Autodesk Fusion 360 part; units mm, degrees
(part 8 of 9)
  spline S368 degree 3 poles (50.2293, -43.6015) (51.1181, -43.6015) (51.7507, -43.8671) (52.1258, -44.3973) knots 0 0 0 0 1 1 1 1
  spline S369 degree 3 poles (52.1258, -44.3973) (52.346, -44.7105) (52.4566, -45.0722) (52.4566, -45.4825) knots 0 0 0 0 1 1 1 1
  spline S370 degree 3 poles (52.4566, -45.4825) (52.4566, -45.961) (52.3201, -46.3538) (52.0483, -46.6607) knots 0 0 0 0 1 1 1 1
  spline S371 degree 3 poles (52.0483, -46.6607) (51.9067, -46.823) (51.7042, -46.9708) (51.4385, -47.1052) knots 0 0 0 0 1 1 1 1
  spline S372 degree 3 poles (51.4385, -47.1052) (51.8282, -47.253) (52.1186, -47.4204) (52.3119, -47.6064) knots 0 0 0 0 1 1 1 1
  spline S373 degree 3 poles (52.3119, -47.6064) (52.6529, -47.9372) (52.8235, -48.394) (52.8235, -48.9758) knots 0 0 0 0 1 1 1 1
  spline S374 degree 3 poles (52.8235, -48.9758) (52.8235, -49.4647) (52.6705, -49.9081) (52.3635, -50.3039) knots 0 0 0 0 1 1 1 1
  spline S375 degree 3 poles (52.3635, -50.3039) (51.9057, -50.8961) (51.1771, -51.1928) (50.1776, -51.1928) knots 0 0 0 0 1 1 1 1
  line L781 (50.1776, -51.1928) -> (46.9685, -51.1928)
  line L782 (46.9685, -51.1928) -> (46.9685, -43.6015)
  line L783 (63.7613, -43.6015) -> (69.2958, -43.6015)
  line L784 (69.2958, -43.6015) -> (69.2958, -44.5317)
  line L785 (69.2958, -44.5317) -> (64.7638, -44.5317)
  line L786 (64.7638, -44.5317) -> (64.7638, -46.8364)
  line L787 (64.7638, -46.8364) -> (68.9548, -46.8364)
  line L788 (68.9548, -46.8364) -> (68.9548, -47.7149)
  line L789 (68.9548, -47.7149) -> (64.7638, -47.7149)
  line L790 (64.7638, -47.7149) -> (64.7638, -50.2884)
  line L791 (64.7638, -50.2884) -> (69.3734, -50.2884)
  line L792 (69.3734, -50.2884) -> (69.3734, -51.1928)
  line L793 (69.3734, -51.1928) -> (63.7613, -51.1928)
  line L794 (63.7613, -51.1928) -> (63.7613, -43.6015)
  line L795 (80.0394, -43.6015) -> (81.2538, -43.6015)
  line L796 (81.2538, -43.6015) -> (85.0882, -49.751)
  line L797 (85.0882, -49.751) -> (85.0882, -43.6015)
  line L798 (85.0882, -43.6015) -> (86.0648, -43.6015)
  line L799 (86.0648, -43.6015) -> (86.0648, -51.1928)
  line L800 (86.0648, -51.1928) -> (84.9125, -51.1928)
  line L801 (84.9125, -51.1928) -> (81.0212, -45.0484)
  line L802 (81.0212, -45.0484) -> (81.0212, -51.1928)
  line L803 (81.0212, -51.1928) -> (80.0394, -51.1928)
  line L804 (80.0394, -51.1928) -> (80.0394, -43.6015)
  line L805 (-86.2575, -62.1017) -> (-80.7229, -62.1017)
  line L806 (-80.7229, -62.1017) -> (-80.7229, -63.0318)
  line L807 (-80.7229, -63.0318) -> (-85.2549, -63.0318)
  line L808 (-85.2549, -63.0318) -> (-85.2549, -65.3366)
  line L809 (-85.2549, -65.3366) -> (-81.064, -65.3366)
  line L810 (-81.064, -65.3366) -> (-81.064, -66.2151)
  line L811 (-81.064, -66.2151) -> (-85.2549, -66.2151)
  line L812 (-85.2549, -66.2151) -> (-85.2549, -68.7886)
  line L813 (-85.2549, -68.7886) -> (-80.6454, -68.7886)
  line L814 (-80.6454, -68.7886) -> (-80.6454, -69.6929)
  line L815 (-80.6454, -69.6929) -> (-86.2575, -69.6929)
  line L816 (-86.2575, -69.6929) -> (-86.2575, -62.1017)
  line L817 (-69.1009, -62.1017) -> (-68.0725, -62.1017)
  line L818 (-68.0725, -62.1017) -> (-68.0725, -68.7886)
  line L819 (-68.0725, -68.7886) -> (-64.2278, -68.7886)
  line L820 (-64.2278, -68.7886) -> (-64.2278, -69.6929)
  line L821 (-64.2278, -69.6929) -> (-69.1009, -69.6929)
  line L822 (-69.1009, -69.6929) -> (-69.1009, -62.1017)
  line L823 (-52.6233, -62.1017) -> (-47.3575, -62.1017)
  line L824 (-47.3575, -62.1017) -> (-47.3575, -63.0318)
  line L825 (-47.3575, -63.0318) -> (-51.595, -63.0318)
  line L826 (-51.595, -63.0318) -> (-51.595, -65.3366)
  line L827 (-51.595, -65.3366) -> (-47.8691, -65.3366)
  line L828 (-47.8691, -65.3366) -> (-47.8691, -66.2409)
  line L829 (-47.8691, -66.2409) -> (-51.595, -66.2409)
  line L830 (-51.595, -66.2409) -> (-51.595, -69.6929)
  line L831 (-51.595, -69.6929) -> (-52.6233, -69.6929)
  line L832 (-52.6233, -69.6929) -> (-52.6233, -62.1017)
  line L833 (-35.7499, -62.1017) -> (-33.5692, -68.5664)
  line L834 (-33.5692, -68.5664) -> (-31.4143, -62.1017)
  line L835 (-31.4143, -62.1017) -> (-30.2619, -62.1017)
  line L836 (-30.2619, -62.1017) -> (-33.0318, -69.6929)
  line L837 (-33.0318, -69.6929) -> (-34.1221, -69.6929)
  line L838 (-34.1221, -69.6929) -> (-36.8868, -62.1017)
  line L839 (-36.8868, -62.1017) -> (-35.7499, -62.1017)
  line L840 (-17.3883, -62.1017) -> (-16.3496, -62.1017)
  line L841 (-16.3496, -62.1017) -> (-16.3496, -69.6929)
  line L842 (-16.3496, -69.6929) -> (-17.3883, -69.6929)
  line L843 (-17.3883, -69.6929) -> (-17.3883, -62.1017)
  line L844 (-2.9137, -62.1017) -> (2.6208, -62.1017)
  line L845 (2.6208, -62.1017) -> (2.6208, -63.0318)
  line L846 (2.6208, -63.0318) -> (-1.9112, -63.0318)
  line L847 (-1.9112, -63.0318) -> (-1.9112, -65.3366)
  line L848 (-1.9112, -65.3366) -> (2.2798, -65.3366)
  line L849 (2.2798, -65.3366) -> (2.2798, -66.2151)
  line L850 (2.2798, -66.2151) -> (-1.9112, -66.2151)
  line L851 (-1.9112, -66.2151) -> (-1.9112, -68.7886)
  line L852 (-1.9112, -68.7886) -> (2.6984, -68.7886)
  line L853 (2.6984, -68.7886) -> (2.6984, -69.6929)
  line L854 (2.6984, -69.6929) -> (-2.9137, -69.6929)
  line L855 (-2.9137, -69.6929) -> (-2.9137, -62.1017)
  spline S376 degree 3 poles (16.8939, -65.5795) (17.3765, -65.5795) (17.7579, -65.4834) (18.038, -65.2901) knots 0 0 0 0 1 1 1 1
  spline S377 degree 3 poles (18.038, -65.2901) (18.3191, -65.0968) (18.4597, -64.7496) (18.4597, -64.2462) knots 0 0 0 0 1 1 1 1
  spline S378 degree 3 poles (18.4597, -64.2462) (18.4597, -63.7057) (18.2633, -63.3367) (17.8706, -63.1404) knots 0 0 0 0 1 1 1 1
  spline S379 degree 3 poles (17.8706, -63.1404) (17.6608, -63.037) (17.3796, -62.9853) (17.0282, -62.9853) knots 0 0 0 0 1 1 1 1
  line L856 (17.0282, -62.9853) -> (14.5168, -62.9853)
  line L857 (14.5168, -62.9853) -> (14.5168, -65.5795)
  line L858 (14.5168, -65.5795) -> (16.8939, -65.5795)
  line L859 (13.4884, -62.1017) -> (17.0024, -62.1017)
  spline S380 degree 3 poles (17.0024, -62.1017) (17.5812, -62.1017) (18.0587, -62.1864) (18.4338, -62.3549) knots 0 0 0 0 1 1 1 1
  spline S381 degree 3 poles (18.4338, -62.3549) (19.147, -62.6784) (19.5035, -63.2768) (19.5035, -64.148) knots 0 0 0 0 1 1 1 1
  spline S382 degree 3 poles (19.5035, -64.148) (19.5035, -64.6028) (19.4095, -64.9749) (19.2224, -65.2643) knots 0 0 0 0 1 1 1 1
  spline S383 degree 3 poles (19.2224, -65.2643) (19.0343, -65.5536) (18.7718, -65.7862) (18.4338, -65.9619) knots 0 0 0 0 1 1 1 1
  spline S384 degree 3 poles (18.4338, -65.9619) (18.7305, -66.0828) (18.9537, -66.2409) (19.1025, -66.4373) knots 0 0 0 0 1 1 1 1
  spline S385 degree 3 poles (19.1025, -66.4373) (19.2524, -66.6337) (19.3361, -66.952) (19.3537, -67.3933) knots 0 0 0 0 1 1 1 1
  line L860 (19.3537, -67.3933) -> (19.3898, -68.4114)
  spline S386 degree 3 poles (19.3898, -68.4114) (19.4002, -68.7007) (19.424, -68.9157) (19.4622, -69.0573) knots 0 0 0 0 1 1 1 1
  spline S387 degree 3 poles (19.4622, -69.0573) (19.5242, -69.2981) (19.6348, -69.4531) (19.7929, -69.5224) knots 0 0 0 0 1 1 1 1
  line L861 (19.7929, -69.5224) -> (19.7929, -69.6929)
  line L862 (19.7929, -69.6929) -> (18.532, -69.6929)
  spline S388 degree 3 poles (18.532, -69.6929) (18.4979, -69.6278) (18.47, -69.5431) (18.4493, -69.4397) knots 0 0 0 0 1 1 1 1
  spline S389 degree 3 poles (18.4493, -69.4397) (18.4287, -69.3364) (18.4111, -69.1369) (18.3977, -68.8403) knots 0 0 0 0 1 1 1 1
  line L863 (18.3977, -68.8403) -> (18.3356, -67.5742)
  spline S390 degree 3 poles (18.3356, -67.5742) (18.3119, -67.0781) (18.1269, -66.7453) (17.7827, -66.5768) knots 0 0 0 0 1 1 1 1
  spline S391 degree 3 poles (17.7827, -66.5768) (17.5863, -66.4838) (17.2783, -66.4373) (16.8577, -66.4373) knots 0 0 0 0 1 1 1 1
  line L864 (16.8577, -66.4373) -> (14.5168, -66.4373)
  line L865 (14.5168, -66.4373) -> (14.5168, -69.6929)
  line L866 (14.5168, -69.6929) -> (13.4884, -69.6929)
  line L867 (13.4884, -69.6929) -> (13.4884, -62.1017)
  line L868 (34.222, -66.582) -> (33.0696, -63.2282)
  line L869 (33.0696, -63.2282) -> (31.8449, -66.582)
  line L870 (31.8449, -66.582) -> (34.222, -66.582)
  line L871 (32.5322, -62.1017) -> (33.6949, -62.1017)
  line L872 (33.6949, -62.1017) -> (36.4493, -69.6929)
  line L873 (36.4493, -69.6929) -> (35.3227, -69.6929)
  line L874 (35.3227, -69.6929) -> (34.5527, -67.4192)
  line L875 (34.5527, -67.4192) -> (31.5503, -67.4192)
  line L876 (31.5503, -67.4192) -> (30.7287, -69.6929)
  line L877 (30.7287, -69.6929) -> (29.6745, -69.6929)
  line L878 (29.6745, -69.6929) -> (32.5322, -62.1017)
  spline S392 degree 3 poles (49.9006, -61.895) (50.8618, -61.895) (51.608, -62.1482) (52.1382, -62.6546) knots 0 0 0 0 1 1 1 1
  spline S393 degree 3 poles (52.1382, -62.6546) (52.6684, -63.161) (52.963, -63.7367) (53.0219, -64.3806) knots 0 0 0 0 1 1 1 1
  line L879 (53.0219, -64.3806) -> (52.0194, -64.3806)
  spline S394 degree 3 poles (52.0194, -64.3806) (51.9057, -63.8917) (51.6793, -63.5042) (51.3403, -63.2179) knots 0 0 0 0 1 1 1 1
  spline S395 degree 3 poles (51.3403, -63.2179) (51.0003, -62.9316) (50.5239, -62.789) (49.911, -62.789) knots 0 0 0 0 1 1 1 1
  spline S396 degree 3 poles (49.911, -62.789) (49.1637, -62.789) (48.5602, -63.0515) (48.0992, -63.5765) knots 0 0 0 0 1 1 1 1
  spline S397 degree 3 poles (48.0992, -63.5765) (47.6393, -64.1026) (47.4098, -64.9077) (47.4098, -65.9929) knots 0 0 0 0 1 1 1 1
  spline S398 degree 3 poles (47.4098, -65.9929) (47.4098, -66.8817) (47.6176, -67.6031) (48.0331, -68.155) knots 0 0 0 0 1 1 1 1
  spline S399 degree 3 poles (48.0331, -68.155) (48.4475, -68.708) (49.0666, -68.985) (49.8903, -68.985) knots 0 0 0 0 1 1 1 1
  spline S400 degree 3 poles (49.8903, -68.985) (50.6479, -68.985) (51.2256, -68.6935) (51.6215, -68.1116) knots 0 0 0 0 1 1 1 1
  spline S401 degree 3 poles (51.6215, -68.1116) (51.8313, -67.8047) (51.9884, -67.4016) (52.0917, -66.9024) knots 0 0 0 0 1 1 1 1
  line L880 (52.0917, -66.9024) -> (53.0942, -66.9024)
  spline S402 degree 3 poles (53.0942, -66.9024) (53.0043, -67.7013) (52.7087, -68.3721) (52.2054, -68.9126) knots 0 0 0 0 1 1 1 1
  spline S403 degree 3 poles (52.2054, -68.9126) (51.6029, -69.5637) (50.7895, -69.8893) (49.7663, -69.8893) knots 0 0 0 0 1 1 1 1
  spline S404 degree 3 poles (49.7663, -69.8893) (48.8847, -69.8893) (48.1436, -69.6226) (47.5442, -69.0883) knots 0 0 0 0 1 1 1 1
  spline S405 degree 3 poles (47.5442, -69.0883) (46.7556, -68.3824) (46.3608, -67.292) (46.3608, -65.8172) knots 0 0 0 0 1 1 1 1
  spline S406 degree 3 poles (46.3608, -65.8172) (46.3608, -64.6979) (46.6574, -63.7791) (47.2496, -63.0628) knots 0 0 0 0 1 1 1 1
  spline S407 degree 3 poles (47.2496, -63.0628) (47.8904, -62.2846) (48.7741, -61.895) (49.9006, -61.895) knots 0 0 0 0 1 1 1 1
  line L881 (63.3965, -62.1017) -> (64.4352, -62.1017)
  line L882 (64.4352, -62.1017) -> (64.4352, -65.2384)
  line L883 (64.4352, -65.2384) -> (68.3832, -65.2384)
  line L884 (68.3832, -65.2384) -> (68.3832, -62.1017)
  line L885 (68.3832, -62.1017) -> (69.4219, -62.1017)
  line L886 (69.4219, -62.1017) -> (69.4219, -69.6929)
  line L887 (69.4219, -69.6929) -> (68.3832, -69.6929)
  line L888 (68.3832, -69.6929) -> (68.3832, -66.1428)
  line L889 (68.3832, -66.1428) -> (64.4352, -66.1428)
  line L890 (64.4352, -66.1428) -> (64.4352, -69.6929)
  line L891 (64.4352, -69.6929) -> (63.3965, -69.6929)
  line L892 (63.3965, -69.6929) -> (63.3965, -62.1017)
  line L893 (86.1527, -62.1017) -> (86.1527, -63.006)
  line L894 (86.1527, -63.006) -> (83.5947, -63.006)
  line L895 (83.5947, -63.006) -> (83.5947, -69.6929)
  line L896 (83.5947, -69.6929) -> (82.5508, -69.6929)
  line L897 (82.5508, -69.6929) -> (82.5508, -63.006)
  line L898 (82.5508, -63.006) -> (79.9929, -63.006)
  line L899 (79.9929, -63.006) -> (79.9929, -62.1017)
  line L900 (79.9929, -62.1017) -> (86.1527, -62.1017)
  spline S408 degree 3 poles (-85.6838, -85.7426) (-85.6601, -86.1736) (-85.5578, -86.5229) (-85.379, -86.7916) knots 0 0 0 0 1 1 1 1
  spline S409 degree 3 poles (-85.379, -86.7916) (-85.0379, -87.295) (-84.4364, -87.5461) (-83.5754, -87.5461) knots 0 0 0 0 1 1 1 1
  spline S410 degree 3 poles (-83.5754, -87.5461) (-83.1899, -87.5461) (-82.8385, -87.4913) (-82.5212, -87.3807) knots 0 0 0 0 1 1 1 1
  spline S411 degree 3 poles (-82.5212, -87.3807) (-81.9084, -87.1668) (-81.6014, -86.7844) (-81.6014, -86.2335) knots 0 0 0 0 1 1 1 1
  spline S412 degree 3 poles (-81.6014, -86.2335) (-81.6014, -85.8201) (-81.7306, -85.5256) (-81.989, -85.3499) knots 0 0 0 0 1 1 1 1
  spline S413 degree 3 poles (-81.989, -85.3499) (-82.2505, -85.1773) (-82.6608, -85.0274) (-83.2189, -84.9003) knots 0 0 0 0 1 1 1 1
  line L901 (-83.2189, -84.9003) -> (-84.2472, -84.6677)
  spline S414 degree 3 poles (-84.2472, -84.6677) (-84.919, -84.5158) (-85.3945, -84.3494) (-85.6735, -84.1665) knots 0 0 0 0 1 1 1 1
  spline S415 degree 3 poles (-85.6735, -84.1665) (-86.1562, -83.8492) (-86.397, -83.3758) (-86.397, -82.7454) knots 0 0 0 0 1 1 1 1
  spline S416 degree 3 poles (-86.397, -82.7454) (-86.397, -82.0632) (-86.1613, -81.5031) (-85.689, -81.0659) knots 0 0 0 0 1 1 1 1
  spline S417 degree 3 poles (-85.689, -81.0659) (-85.2167, -80.6287) (-84.549, -80.4096) (-83.684, -80.4096) knots 0 0 0 0 1 1 1 1
  spline S418 degree 3 poles (-83.684, -80.4096) (-82.8882, -80.4096) (-82.2122, -80.6018) (-81.6552, -80.9863) knots 0 0 0 0 1 1 1 1
  spline S419 degree 3 poles (-81.6552, -80.9863) (-81.0991, -81.3697) (-80.8211, -81.9837) (-80.8211, -82.828) knots 0 0 0 0 1 1 1 1
  line L902 (-80.8211, -82.828) -> (-81.7874, -82.828)
  spline S420 degree 3 poles (-81.7874, -82.828) (-81.8391, -82.4219) (-81.9497, -82.1097) (-82.1182, -81.8927) knots 0 0 0 0 1 1 1 1
  spline S421 degree 3 poles (-82.1182, -81.8927) (-82.4313, -81.4969) (-82.9636, -81.2984) (-83.715, -81.2984) knots 0 0 0 0 1 1 1 1
  spline S422 degree 3 poles (-83.715, -81.2984) (-84.3217, -81.2984) (-84.7568, -81.4255) (-85.0224, -81.6808) knots 0 0 0 0 1 1 1 1
  spline S423 degree 3 poles (-85.0224, -81.6808) (-85.288, -81.9361) (-85.4203, -82.2317) (-85.4203, -82.5697) knots 0 0 0 0 1 1 1 1
  spline S424 degree 3 poles (-85.4203, -82.5697) (-85.4203, -82.9417) (-85.2653, -83.2135) (-84.9552, -83.3861) knots 0 0 0 0 1 1 1 1
  spline S425 degree 3 poles (-84.9552, -83.3861) (-84.7516, -83.4967) (-84.2917, -83.6342) (-83.5754, -83.7996) knots 0 0 0 0 1 1 1 1
  line L903 (-83.5754, -83.7996) -> (-82.5109, -84.0424)
  spline S426 degree 3 poles (-82.5109, -84.0424) (-81.9972, -84.1592) (-81.6014, -84.3194) (-81.3224, -84.523) knots 0 0 0 0 1 1 1 1
  spline S427 degree 3 poles (-81.3224, -84.523) (-80.8397, -84.8775) (-80.5989, -85.3933) (-80.5989, -86.0682) knots 0 0 0 0 1 1 1 1
  spline S428 degree 3 poles (-80.5989, -86.0682) (-80.5989, -86.9084) (-80.9048, -87.5099) (-81.5167, -87.8717) knots 0 0 0 0 1 1 1 1
  spline S429 degree 3 poles (-81.5167, -87.8717) (-82.1275, -88.2334) (-82.8385, -88.4143) (-83.6478, -88.4143) knots 0 0 0 0 1 1 1 1
  spline S430 degree 3 poles (-83.6478, -88.4143) (-84.5914, -88.4143) (-85.3304, -88.1735) (-85.8647, -87.6908) knots 0 0 0 0 1 1 1 1
  spline S431 degree 3 poles (-85.8647, -87.6908) (-86.399, -87.2123) (-86.6605, -86.5622) (-86.6502, -85.7426) knots 0 0 0 0 1 1 1 1
  line L904 (-86.6502, -85.7426) -> (-85.6838, -85.7426)
  line L905 (-69.5887, -80.6008) -> (-64.0542, -80.6008)
  line L906 (-64.0542, -80.6008) -> (-64.0542, -81.531)
  line L907 (-64.0542, -81.531) -> (-68.5862, -81.531)
  line L908 (-68.5862, -81.531) -> (-68.5862, -83.8357)
  line L909 (-68.5862, -83.8357) -> (-64.3952, -83.8357)
  line L910 (-64.3952, -83.8357) -> (-64.3952, -84.7142)
  line L911 (-64.3952, -84.7142) -> (-68.5862, -84.7142)
  line L912 (-68.5862, -84.7142) -> (-68.5862, -87.2877)
  line L913 (-68.5862, -87.2877) -> (-63.9766, -87.2877)
  line L914 (-63.9766, -87.2877) -> (-63.9766, -88.1921)
  line L915 (-63.9766, -88.1921) -> (-69.5887, -88.1921)
  line L916 (-69.5887, -88.1921) -> (-69.5887, -80.6008)
  spline S432 degree 3 poles (-50.1119, -80.3941) (-49.1507, -80.3941) (-48.4045, -80.6473) (-47.8743, -81.1537) knots 0 0 0 0 1 1 1 1
  spline S433 degree 3 poles (-47.8743, -81.1537) (-47.3441, -81.6602) (-47.0495, -82.2358) (-46.9906, -82.8797) knots 0 0 0 0 1 1 1 1
  line L917 (-46.9906, -82.8797) -> (-47.9931, -82.8797)
  spline S434 degree 3 poles (-47.9931, -82.8797) (-48.1068, -82.3909) (-48.3332, -82.0033) (-48.6722, -81.717) knots 0 0 0 0 1 1 1 1
  spline S435 degree 3 poles (-48.6722, -81.717) (-49.0122, -81.4307) (-49.4886, -81.2881) (-50.1015, -81.2881) knots 0 0 0 0 1 1 1 1
  spline S436 degree 3 poles (-50.1015, -81.2881) (-50.8488, -81.2881) (-51.4523, -81.5506) (-51.9133, -82.0756) knots 0 0 0 0 1 1 1 1
  spline S437 degree 3 poles (-51.9133, -82.0756) (-52.3732, -82.6017) (-52.6027, -83.4068) (-52.6027, -84.492) knots 0 0 0 0 1 1 1 1
  spline S438 degree 3 poles (-52.6027, -84.492) (-52.6027, -85.3809) (-52.3949, -86.1023) (-51.9794, -86.6542) knots 0 0 0 0 1 1 1 1
  spline S439 degree 3 poles (-51.9794, -86.6542) (-51.565, -87.2071) (-50.9459, -87.4841) (-50.1222, -87.4841) knots 0 0 0 0 1 1 1 1
  spline S440 degree 3 poles (-50.1222, -87.4841) (-49.3646, -87.4841) (-48.7869, -87.1926) (-48.391, -86.6108) knots 0 0 0 0 1 1 1 1
  spline S441 degree 3 poles (-48.391, -86.6108) (-48.1812, -86.3038) (-48.0241, -85.9007) (-47.9208, -85.4015) knots 0 0 0 0 1 1 1 1
  line L918 (-47.9208, -85.4015) -> (-46.9183, -85.4015)
  spline S442 degree 3 poles (-46.9183, -85.4015) (-47.0082, -86.2004) (-47.3038, -86.8712) (-47.8071, -87.4117) knots 0 0 0 0 1 1 1 1
  spline S443 degree 3 poles (-47.8071, -87.4117) (-48.4096, -88.0629) (-49.223, -88.3884) (-50.2462, -88.3884) knots 0 0 0 0 1 1 1 1
  spline S444 degree 3 poles (-50.2462, -88.3884) (-51.1278, -88.3884) (-51.8689, -88.1218) (-52.4683, -87.5874) knots 0 0 0 0 1 1 1 1
  spline S445 degree 3 poles (-52.4683, -87.5874) (-53.2569, -86.8815) (-53.6517, -85.7912) (-53.6517, -84.3163) knots 0 0 0 0 1 1 1 1
  spline S446 degree 3 poles (-53.6517, -84.3163) (-53.6517, -83.197) (-53.3551, -82.2782) (-52.7629, -81.562) knots 0 0 0 0 1 1 1 1
  spline S447 degree 3 poles (-52.7629, -81.562) (-52.1221, -80.7837) (-51.2384, -80.3941) (-50.1119, -80.3941) knots 0 0 0 0 1 1 1 1
  line L919 (-36.616, -80.6008) -> (-35.5773, -80.6008)
  line L920 (-35.5773, -80.6008) -> (-35.5773, -83.7375)
  line L921 (-35.5773, -83.7375) -> (-31.6293, -83.7375)
  line L922 (-31.6293, -83.7375) -> (-31.6293, -80.6008)
  line L923 (-31.6293, -80.6008) -> (-30.5906, -80.6008)
  line L924 (-30.5906, -80.6008) -> (-30.5906, -88.1921)
  line L925 (-30.5906, -88.1921) -> (-31.6293, -88.1921)
  line L926 (-31.6293, -88.1921) -> (-31.6293, -84.6419)
  line L927 (-31.6293, -84.6419) -> (-35.5773, -84.6419)
  line L928 (-35.5773, -84.6419) -> (-35.5773, -88.1921)
  line L929 (-35.5773, -88.1921) -> (-36.616, -88.1921)
  line L930 (-36.616, -88.1921) -> (-36.616, -80.6008)
  spline S448 degree 3 poles (-19.0088, -85.7426) (-18.9851, -86.1736) (-18.8828, -86.5229) (-18.704, -86.7916) knots 0 0 0 0 1 1 1 1
  spline S449 degree 3 poles (-18.704, -86.7916) (-18.3629, -87.295) (-17.7614, -87.5461) (-16.9004, -87.5461) knots 0 0 0 0 1 1 1 1
  spline S450 degree 3 poles (-16.9004, -87.5461) (-16.5149, -87.5461) (-16.1635, -87.4913) (-15.8462, -87.3807) knots 0 0 0 0 1 1 1 1
  spline S451 degree 3 poles (-15.8462, -87.3807) (-15.2334, -87.1668) (-14.9264, -86.7844) (-14.9264, -86.2335) knots 0 0 0 0 1 1 1 1
  spline S452 degree 3 poles (-14.9264, -86.2335) (-14.9264, -85.8201) (-15.0556, -85.5256) (-15.314, -85.3499) knots 0 0 0 0 1 1 1 1
  spline S453 degree 3 poles (-15.314, -85.3499) (-15.5755, -85.1773) (-15.9858, -85.0274) (-16.5439, -84.9003) knots 0 0 0 0 1 1 1 1
  line L931 (-16.5439, -84.9003) -> (-17.5722, -84.6677)
  spline S454 degree 3 poles (-17.5722, -84.6677) (-18.244, -84.5158) (-18.7195, -84.3494) (-18.9985, -84.1665) knots 0 0 0 0 1 1 1 1
  spline S455 degree 3 poles (-18.9985, -84.1665) (-19.4812, -83.8492) (-19.722, -83.3758) (-19.722, -82.7454) knots 0 0 0 0 1 1 1 1
  spline S456 degree 3 poles (-19.722, -82.7454) (-19.722, -82.0632) (-19.4863, -81.5031) (-19.014, -81.0659) knots 0 0 0 0 1 1 1 1
  spline S457 degree 3 poles (-19.014, -81.0659) (-18.5417, -80.6287) (-17.874, -80.4096) (-17.009, -80.4096) knots 0 0 0 0 1 1 1 1
  spline S458 degree 3 poles (-17.009, -80.4096) (-16.2132, -80.4096) (-15.5372, -80.6018) (-14.9802, -80.9863) knots 0 0 0 0 1 1 1 1
  spline S459 degree 3 poles (-14.9802, -80.9863) (-14.4241, -81.3697) (-14.1461, -81.9837) (-14.1461, -82.828) knots 0 0 0 0 1 1 1 1
  line L932 (-14.1461, -82.828) -> (-15.1124, -82.828)
  spline S460 degree 3 poles (-15.1124, -82.828) (-15.1641, -82.4219) (-15.2747, -82.1097) (-15.4432, -81.8927) knots 0 0 0 0 1 1 1 1
  spline S461 degree 3 poles (-15.4432, -81.8927) (-15.7563, -81.4969) (-16.2886, -81.2984) (-17.04, -81.2984) knots 0 0 0 0 1 1 1 1
  spline S462 degree 3 poles (-17.04, -81.2984) (-17.6467, -81.2984) (-18.0818, -81.4255) (-18.3474, -81.6808) knots 0 0 0 0 1 1 1 1
  spline S463 degree 3 poles (-18.3474, -81.6808) (-18.613, -81.9361) (-18.7453, -82.2317) (-18.7453, -82.5697) knots 0 0 0 0 1 1 1 1
  spline S464 degree 3 poles (-18.7453, -82.5697) (-18.7453, -82.9417) (-18.5903, -83.2135) (-18.2802, -83.3861) knots 0 0 0 0 1 1 1 1
  spline S465 degree 3 poles (-18.2802, -83.3861) (-18.0766, -83.4967) (-17.6167, -83.6342) (-16.9004, -83.7996) knots 0 0 0 0 1 1 1 1
  line L933 (-16.9004, -83.7996) -> (-15.8359, -84.0424)
  spline S466 degree 3 poles (-15.8359, -84.0424) (-15.3222, -84.1592) (-14.9264, -84.3194) (-14.6474, -84.523) knots 0 0 0 0 1 1 1 1
  spline S467 degree 3 poles (-14.6474, -84.523) (-14.1647, -84.8775) (-13.9239, -85.3933) (-13.9239, -86.0682) knots 0 0 0 0 1 1 1 1
  spline S468 degree 3 poles (-13.9239, -86.0682) (-13.9239, -86.9084) (-14.2298, -87.5099) (-14.8417, -87.8717) knots 0 0 0 0 1 1 1 1
  spline S469 degree 3 poles (-14.8417, -87.8717) (-15.4525, -88.2334) (-16.1635, -88.4143) (-16.9728, -88.4143) knots 0 0 0 0 1 1 1 1
  spline S470 degree 3 poles (-16.9728, -88.4143) (-17.9164, -88.4143) (-18.6554, -88.1735) (-19.1897, -87.6908) knots 0 0 0 0 1 1 1 1
  spline S471 degree 3 poles (-19.1897, -87.6908) (-19.724, -87.2123) (-19.9855, -86.5622) (-19.9752, -85.7426) knots 0 0 0 0 1 1 1 1
  line L934 (-19.9752, -85.7426) -> (-19.0088, -85.7426)
  line L935 (-0.7195, -80.6008) -> (0.3192, -80.6008)
  line L936 (0.3192, -80.6008) -> (0.3192, -88.1921)
  line L937 (0.3192, -88.1921) -> (-0.7195, -88.1921)
  line L938 (-0.7195, -88.1921) -> (-0.7195, -80.6008)
  line L939 (14.4806, -80.6008) -> (14.4806, -85.293)
  spline S472 degree 3 poles (14.4806, -85.293) (14.4806, -85.8439) (14.5839, -86.3028) (14.7906, -86.6676) knots 0 0 0 0 1 1 1 1
  spline S473 degree 3 poles (14.7906, -86.6676) (15.0976, -87.2185) (15.6144, -87.4944) (16.3409, -87.4944) knots 0 0 0 0 1 1 1 1
  spline S474 degree 3 poles (16.3409, -87.4944) (17.2122, -87.4944) (17.8054, -87.1968) (18.1186, -86.6004) knots 0 0 0 0 1 1 1 1
  spline S475 degree 3 poles (18.1186, -86.6004) (18.2871, -86.2769) (18.3718, -85.8408) (18.3718, -85.293) knots 0 0 0 0 1 1 1 1
  line L940 (18.3718, -85.293) -> (18.3718, -80.6008)
  line L941 (18.3718, -80.6008) -> (19.4157, -80.6008)
  line L942 (19.4157, -80.6008) -> (19.4157, -84.8641)
  spline S476 degree 3 poles (19.4157, -84.8641) (19.4157, -85.7974) (19.2896, -86.5157) (19.0384, -87.019) knots 0 0 0 0 1 1 1 1
  spline S477 degree 3 poles (19.0384, -87.019) (18.5765, -87.9357) (17.7052, -88.3936) (16.4236, -88.3936) knots 0 0 0 0 1 1 1 1
  spline S478 degree 3 poles (16.4236, -88.3936) (15.142, -88.3936) (14.2718, -87.9357) (13.814, -87.019) knots 0 0 0 0 1 1 1 1
  spline S479 degree 3 poles (13.814, -87.019) (13.5628, -86.5157) (13.4367, -85.7974) (13.4367, -84.8641) knots 0 0 0 0 1 1 1 1
  line L943 (13.4367, -84.8641) -> (13.4367, -80.6008)
  line L944 (13.4367, -80.6008) -> (14.4806, -80.6008)
  line L945 (30.059, -80.6008) -> (31.0977, -80.6008)
  line L946 (31.0977, -80.6008) -> (31.0977, -83.7375)
  line L947 (31.0977, -83.7375) -> (35.0457, -83.7375)
  line L948 (35.0457, -83.7375) -> (35.0457, -80.6008)
  line L949 (35.0457, -80.6008) -> (36.0844, -80.6008)
  line L950 (36.0844, -80.6008) -> (36.0844, -88.1921)
  line L951 (36.0844, -88.1921) -> (35.0457, -88.1921)
  line L952 (35.0457, -88.1921) -> (35.0457, -84.6419)
  line L953 (35.0457, -84.6419) -> (31.0977, -84.6419)
  line L954 (31.0977, -84.6419) -> (31.0977, -88.1921)
  line L955 (31.0977, -88.1921) -> (30.059, -88.1921)
  line L956 (30.059, -88.1921) -> (30.059, -80.6008)
  spline S480 degree 3 poles (50.2314, -84.0786) (50.714, -84.0786) (51.0954, -83.9825) (51.3755, -83.7892) knots 0 0 0 0 1 1 1 1
  spline S481 degree 3 poles (51.3755, -83.7892) (51.6566, -83.596) (51.7972, -83.2487) (51.7972, -82.7454) knots 0 0 0 0 1 1 1 1
  spline S482 degree 3 poles (51.7972, -82.7454) (51.7972, -82.2048) (51.6008, -81.8359) (51.2081, -81.6395) knots 0 0 0 0 1 1 1 1
  spline S483 degree 3 poles (51.2081, -81.6395) (50.9983, -81.5361) (50.7171, -81.4845) (50.3657, -81.4845) knots 0 0 0 0 1 1 1 1
  line L957 (50.3657, -81.4845) -> (47.8543, -81.4845)
  line L958 (47.8543, -81.4845) -> (47.8543, -84.0786)
  line L959 (47.8543, -84.0786) -> (50.2314, -84.0786)
  line L960 (46.8259, -80.6008) -> (50.3399, -80.6008)
  spline S484 degree 3 poles (50.3399, -80.6008) (50.9187, -80.6008) (51.3962, -80.6855) (51.7713, -80.854) knots 0 0 0 0 1 1 1 1
  spline S485 degree 3 poles (51.7713, -80.854) (52.4845, -81.1775) (52.841, -81.7759) (52.841, -82.6472) knots 0 0 0 0 1 1 1 1
  spline S486 degree 3 poles (52.841, -82.6472) (52.841, -83.1019) (52.747, -83.474) (52.5599, -83.7634) knots 0 0 0 0 1 1 1 1
  spline S487 degree 3 poles (52.5599, -83.7634) (52.3718, -84.0528) (52.1093, -84.2853) (51.7713, -84.461) knots 0 0 0 0 1 1 1 1
  spline S488 degree 3 poles (51.7713, -84.461) (52.068, -84.5819) (52.2912, -84.7401) (52.44, -84.9364) knots 0 0 0 0 1 1 1 1
  spline S489 degree 3 poles (52.44, -84.9364) (52.5899, -85.1328) (52.6736, -85.4511) (52.6912, -85.8925) knots 0 0 0 0 1 1 1 1
  line L961 (52.6912, -85.8925) -> (52.7273, -86.9105)
  spline S490 degree 3 poles (52.7273, -86.9105) (52.7377, -87.1999) (52.7615, -87.4148) (52.7997, -87.5564) knots 0 0 0 0 1 1 1 1
  spline S491 degree 3 poles (52.7997, -87.5564) (52.8617, -87.7972) (52.9723, -87.9523) (53.1304, -88.0215) knots 0 0 0 0 1 1 1 1
  line L962 (53.1304, -88.0215) -> (53.1304, -88.1921)
  line L963 (53.1304, -88.1921) -> (51.8695, -88.1921)
  spline S492 degree 3 poles (51.8695, -88.1921) (51.8354, -88.1269) (51.8075, -88.0422) (51.7868, -87.9388) knots 0 0 0 0 1 1 1 1
  spline S493 degree 3 poles (51.7868, -87.9388) (51.7662, -87.8355) (51.7486, -87.636) (51.7352, -87.3394) knots 0 0 0 0 1 1 1 1
  line L964 (51.7352, -87.3394) -> (51.6731, -86.0733)
  spline S494 degree 3 poles (51.6731, -86.0733) (51.6494, -85.5772) (51.4644, -85.2444) (51.1202, -85.076) knots 0 0 0 0 1 1 1 1
  spline S495 degree 3 poles (51.1202, -85.076) (50.9238, -84.983) (50.6158, -84.9364) (50.1952, -84.9364) knots 0 0 0 0 1 1 1 1
  line L965 (50.1952, -84.9364) -> (47.8543, -84.9364)
  line L966 (47.8543, -84.9364) -> (47.8543, -88.1921)
  line L967 (47.8543, -88.1921) -> (46.8259, -88.1921)
  line L968 (46.8259, -88.1921) -> (46.8259, -80.6008)
  line L969 (63.074, -80.6008) -> (64.2729, -80.6008)
  line L970 (64.2729, -80.6008) -> (66.4536, -84.2491)
  line L971 (66.4536, -84.2491) -> (68.6344, -80.6008)
  line L972 (68.6344, -80.6008) -> (69.8384, -80.6008)
  line L973 (69.8384, -80.6008) -> (66.9704, -85.1328)
  line L974 (66.9704, -85.1328) -> (66.9704, -88.1921)
  line L975 (66.9704, -88.1921) -> (65.942, -88.1921)
  line L976 (65.942, -88.1921) -> (65.942, -85.1328)
  line L977 (65.942, -85.1328) -> (63.074, -80.6008)
  line L978 (80.43, -80.6008) -> (85.9646, -80.6008)
  line L979 (85.9646, -80.6008) -> (85.9646, -81.531)
  line L980 (85.9646, -81.531) -> (81.4326, -81.531)
  line L981 (81.4326, -81.531) -> (81.4326, -83.8357)
  line L982 (81.4326, -83.8357) -> (85.6235, -83.8357)
  line L983 (85.6235, -83.8357) -> (85.6235, -84.7142)
  line L984 (85.6235, -84.7142) -> (81.4326, -84.7142)
  line L985 (81.4326, -84.7142) -> (81.4326, -87.2877)
  line L986 (81.4326, -87.2877) -> (86.0421, -87.2877)
  line L987 (86.0421, -87.2877) -> (86.0421, -88.1921)
  line L988 (86.0421, -88.1921) -> (80.43, -88.1921)
  line L989 (80.43, -88.1921) -> (80.43, -80.6008)
sketch "Sketch8" plane through (0, 0, 0) normal (0, 0, 1) x (1, 0, 0)
  line L0 (-150, 150) -> (150, 150)
  line L1 (150, 150) -> (150, -150)
  line L2 (150, -150) -> (-150, -150)
  line L3 (-150, -150) -> (-150, 150)
  spline S0 degree 3 poles (102.2213, -100.0075) (102.2213, -101.2499) (101.2142, -102.2576) (99.9715, -102.2576) knots 0 0 0 0 1 1 1 1
  spline S1 degree 3 poles (99.9715, -102.2576) (98.7292, -102.2576) (97.7218, -101.2502) (97.7218, -100.0075) knots 0 0 0 0 1 1 1 1
  spline S2 degree 3 poles (97.7218, -100.0075) (97.7218, -98.7648) (98.7292, -97.7574) (99.9715, -97.7574) knots 0 0 0 0 1 1 1 1
  spline S3 degree 3 poles (99.9715, -97.7574) (101.2142, -97.7577) (102.2213, -98.7652) (102.2213, -100.0075) knots 0 0 0 0 1 1 1 1
  circle A0 centre (99.9716, -100.0075) radius 2.2497
  spline S4 degree 3 poles (-97.7546, -100.0075) (-97.7546, -101.2499) (-98.7617, -102.2576) (-100.0043, -102.2576) knots 0 0 0 0 1 1 1 1
  spline S5 degree 3 poles (-100.0043, -102.2576) (-101.2467, -102.2576) (-102.2541, -101.2502) (-102.2541, -100.0075) knots 0 0 0 0 1 1 1 1
  spline S6 degree 3 poles (-102.2541, -100.0075) (-102.2541, -98.7648) (-101.2467, -97.7574) (-100.0043, -97.7574) knots 0 0 0 0 1 1 1 1
  spline S7 degree 3 poles (-100.0043, -97.7574) (-98.7617, -97.7577) (-97.7546, -98.7652) (-97.7546, -100.0075) knots 0 0 0 0 1 1 1 1
  circle A1 centre (-100.0044, -100.0075) radius 2.2497
  spline S8 degree 3 poles (-97.7546, 99.9677) (-97.7546, 98.7254) (-98.7617, 97.7179) (-100.0043, 97.7179) knots 0 0 0 0 1 1 1 1
  spline S9 degree 3 poles (-100.0043, 97.7179) (-101.2467, 97.7179) (-102.2541, 98.7254) (-102.2541, 99.9677) knots 0 0 0 0 1 1 1 1
  spline S10 degree 3 poles (-102.2541, 99.9677) (-102.2541, 101.21) (-101.2467, 102.2175) (-100.0043, 102.2175) knots 0 0 0 0 1 1 1 1
  spline S11 degree 3 poles (-100.0043, 102.2175) (-98.7617, 102.2175) (-97.7546, 101.21) (-97.7546, 99.9677) knots 0 0 0 0 1 1 1 1
  circle A2 centre (-100.0044, 99.9677) radius 2.2497
  spline S12 degree 3 poles (102.2213, 99.9677) (102.2213, 98.7254) (101.2142, 97.7179) (99.9715, 97.7179) knots 0 0 0 0 1 1 1 1
  spline S13 degree 3 poles (99.9715, 97.7179) (98.7292, 97.7179) (97.7218, 98.7254) (97.7218, 99.9677) knots 0 0 0 0 1 1 1 1
  spline S14 degree 3 poles (97.7218, 99.9677) (97.7218, 101.21) (98.7292, 102.2175) (99.9715, 102.2175) knots 0 0 0 0 1 1 1 1
  spline S15 degree 3 poles (99.9715, 102.2175) (101.2142, 102.2175) (102.2213, 101.21) (102.2213, 99.9677) knots 0 0 0 0 1 1 1 1
  circle A3 centre (99.9716, 99.9677) radius 2.2497
  line L4 (-86.6323, 79.2853) -> (-80.9789, 79.2853) construction
  line L5 (-80.9789, 79.2853) -> (-80.9789, 89.8687) construction
  line L6 (-80.9789, 89.8687) -> (-86.6323, 89.8687) construction
  line L7 (-86.6323, 89.8687) -> (-86.6323, 79.2853) construction
  line L8 (-69.9635, 79.2853) -> (-63.9329, 79.2853) construction
  line L9 (-63.9329, 79.2853) -> (-63.9329, 89.8687) construction
  line L10 (-63.9329, 89.8687) -> (-69.9635, 89.8687) construction
  line L11 (-69.9635, 89.8687) -> (-69.9635, 79.2853) construction
  line L12 (-53.2948, 79.2853) -> (-47.0316, 79.2853) construction
  line L13 (-47.0316, 79.2853) -> (-47.0316, 89.8687) construction
  line L14 (-47.0316, 89.8687) -> (-53.2948, 89.8687) construction
  line L15 (-53.2948, 89.8687) -> (-53.2948, 79.2853) construction
  line L16 (-36.626, 79.2853) -> (-35.6235, 79.2853) construction
  line L17 (-35.6235, 79.2853) -> (-35.6235, 89.8687) construction
  line L18 (-35.6235, 89.8687) -> (-36.626, 89.8687) construction
  line L19 (-36.626, 89.8687) -> (-36.626, 79.2853) construction
  line L20 (-19.9573, 79.2853) -> (-13.9267, 79.2853) construction
  line L21 (-13.9267, 79.2853) -> (-13.9267, 89.8687) construction
  line L22 (-13.9267, 89.8687) -> (-19.9573, 89.8687) construction
  line L23 (-19.9573, 89.8687) -> (-19.9573, 79.2853) construction
  line L24 (-3.2885, 79.2853) -> (2.7163, 79.2853) construction
  line L25 (2.7163, 79.2853) -> (2.7163, 89.8687) construction
  line L26 (2.7163, 89.8687) -> (-3.2885, 89.8687) construction
  line L27 (-3.2885, 89.8687) -> (-3.2885, 79.2853) construction
  line L28 (13.3802, 79.2853) -> (18.1138, 79.2853) construction
  line L29 (18.1138, 79.2853) -> (18.1138, 89.8687) construction
  line L30 (18.1138, 89.8687) -> (13.3802, 89.8687) construction
  line L31 (13.3802, 89.8687) -> (13.3802, 79.2853) construction
  line L32 (30.049, 79.2853) -> (35.1598, 79.2853) construction
  line L33 (35.1598, 79.2853) -> (35.1598, 89.8687) construction
  line L34 (35.1598, 89.8687) -> (30.049, 89.8687) construction
  line L35 (30.049, 89.8687) -> (30.049, 79.2853) construction
  line L36 (46.7177, 79.2853) -> (52.676, 79.2853) construction
  line L37 (52.676, 79.2853) -> (52.676, 89.8687) construction
  line L38 (52.676, 89.8687) -> (46.7177, 89.8687) construction
  line L39 (46.7177, 89.8687) -> (46.7177, 79.2853) construction
  line L40 (63.3865, 79.2853) -> (69.3551, 79.2853) construction
  line L41 (69.3551, 79.2853) -> (69.3551, 89.8687) construction
  line L42 (69.3551, 89.8687) -> (63.3865, 89.8687) construction
  line L43 (63.3865, 89.8687) -> (63.3865, 79.2853) construction
  line L44 (80.0552, 79.2853) -> (85.166, 79.2853) construction
  line L45 (85.166, 79.2853) -> (85.166, 89.8687) construction
  line L46 (85.166, 89.8687) -> (80.0552, 89.8687) construction
  line L47 (80.0552, 89.8687) -> (80.0552, 79.2853) construction
  line L48 (-86.6323, 60.7853) -> (-80.643, 60.7853) construction
  line L49 (-80.643, 60.7853) -> (-80.643, 71.3687) construction
  line L50 (-80.643, 71.3687) -> (-86.6323, 71.3687) construction
  line L51 (-86.6323, 71.3687) -> (-86.6323, 60.7853) construction
  line L52 (-69.9635, 60.7853) -> (-64.3101, 60.7853) construction
  line L53 (-64.3101, 60.7853) -> (-64.3101, 71.3687) construction
  line L54 (-64.3101, 71.3687) -> (-69.9635, 71.3687) construction
  line L55 (-69.9635, 71.3687) -> (-69.9635, 60.7853) construction
  line L56 (-53.2948, 60.7853) -> (-47.352, 60.7853) construction
  line L57 (-47.352, 60.7853) -> (-47.352, 71.3687) construction
  line L58 (-47.352, 71.3687) -> (-53.2948, 71.3687) construction
  line L59 (-53.2948, 71.3687) -> (-53.2948, 60.7853) construction
  line L60 (-36.626, 60.7853) -> (-30.6574, 60.7853) construction
  line L61 (-30.6574, 60.7853) -> (-30.6574, 71.3687) construction
  line L62 (-30.6574, 71.3687) -> (-36.626, 71.3687) construction
  line L63 (-36.626, 71.3687) -> (-36.626, 60.7853) construction
  line L64 (-19.9573, 60.7853) -> (-13.968, 60.7853) construction
  line L65 (-13.968, 60.7853) -> (-13.968, 71.3687) construction
  line L66 (-13.968, 71.3687) -> (-19.9573, 71.3687) construction
  line L67 (-19.9573, 71.3687) -> (-19.9573, 60.7853) construction
  line L68 (-3.2885, 60.7853) -> (6.4525, 60.7853) construction
  line L69 (6.4525, 60.7853) -> (6.4525, 71.3687) construction
  line L70 (6.4525, 71.3687) -> (-3.2885, 71.3687) construction
  line L71 (-3.2885, 71.3687) -> (-3.2885, 60.7853) construction
  line L72 (13.3802, 60.7853) -> (20.4702, 60.7853) construction
  line L73 (20.4702, 60.7853) -> (20.4702, 71.3687) construction
  line L74 (20.4702, 71.3687) -> (13.3802, 71.3687) construction
  line L75 (13.3802, 71.3687) -> (13.3802, 60.7853) construction
  line L76 (30.049, 60.7853) -> (36.0176, 60.7853) construction
  line L77 (36.0176, 60.7853) -> (36.0176, 71.3687) construction
  line L78 (36.0176, 71.3687) -> (30.049, 71.3687) construction
  line L79 (30.049, 71.3687) -> (30.049, 60.7853) construction
  line L80 (46.7177, 60.7853) -> (52.707, 60.7853) construction
  line L81 (52.707, 60.7853) -> (52.707, 71.3687) construction
  line L82 (52.707, 71.3687) -> (46.7177, 71.3687) construction
  line L83 (46.7177, 71.3687) -> (46.7177, 60.7853) construction
  line L84 (63.3865, 60.7853) -> (64.389, 60.7853) construction
  line L85 (64.389, 60.7853) -> (64.389, 71.3687) construction
  line L86 (64.389, 71.3687) -> (63.3865, 71.3687) construction
  line L87 (63.3865, 71.3687) -> (63.3865, 60.7853) construction
  line L88 (80.0552, 60.7853) -> (87.0625, 60.7853) construction
  line L89 (87.0625, 60.7853) -> (87.0625, 71.3687) construction
  line L90 (87.0625, 71.3687) -> (80.0552, 71.3687) construction
  line L91 (80.0552, 71.3687) -> (80.0552, 60.7853) construction
  line L92 (-86.6323, 42.2853) -> (-80.3691, 42.2853) construction
  line L93 (-80.3691, 42.2853) -> (-80.3691, 52.8686) construction
  line L94 (-80.3691, 52.8686) -> (-86.6323, 52.8686) construction
  line L95 (-86.6323, 52.8686) -> (-86.6323, 42.2853) construction
  line L96 (-69.9635, 42.2853) -> (-63.2869, 42.2853) construction
  line L97 (-63.2869, 42.2853) -> (-63.2869, 52.8686) construction
  line L98 (-63.2869, 52.8686) -> (-69.9635, 52.8686) construction
  line L99 (-69.9635, 52.8686) -> (-69.9635, 42.2853) construction
  line L100 (-53.2948, 42.2853) -> (-47.6414, 42.2853) construction
  line L101 (-47.6414, 42.2853) -> (-47.6414, 52.8686) construction
  line L102 (-47.6414, 52.8686) -> (-53.2948, 52.8686) construction
  line L103 (-53.2948, 52.8686) -> (-53.2948, 42.2853) construction
  line L104 (-36.626, 42.2853) -> (-35.6235, 42.2853) construction
  line L105 (-35.6235, 42.2853) -> (-35.6235, 52.8686) construction
  line L106 (-35.6235, 52.8686) -> (-36.626, 52.8686) construction
  line L107 (-36.626, 52.8686) -> (-36.626, 42.2853) construction
  line L108 (-19.9573, 42.2853) -> (-13.0275, 42.2853) construction
  line L109 (-13.0275, 42.2853) -> (-13.0275, 52.8686) construction
  line L110 (-13.0275, 52.8686) -> (-19.9573, 52.8686) construction
  line L111 (-19.9573, 52.8686) -> (-19.9573, 42.2853) construction
  line L112 (-3.2885, 42.2853) -> (-2.286, 42.2853) construction
  line L113 (-2.286, 42.2853) -> (-2.286, 52.8686) construction
  line L114 (-2.286, 52.8686) -> (-3.2885, 52.8686) construction
  line L115 (-3.2885, 52.8686) -> (-3.2885, 42.2853) construction
  line L116 (13.3802, 42.2853) -> (19.0336, 42.2853) construction
  line L117 (19.0336, 42.2853) -> (19.0336, 52.8686) construction
  line L118 (19.0336, 52.8686) -> (13.3802, 52.8686) construction
  line L119 (13.3802, 52.8686) -> (13.3802, 42.2853) construction
  line L120 (30.049, 42.2853) -> (36.7256, 42.2853) construction
  line L121 (36.7256, 42.2853) -> (36.7256, 52.8686) construction
  line L122 (36.7256, 52.8686) -> (30.049, 52.8686) construction
  line L123 (30.049, 52.8686) -> (30.049, 42.2853) construction
  line L124 (46.7177, 42.2853) -> (52.7225, 42.2853) construction
  line L125 (52.7225, 42.2853) -> (52.7225, 52.8686) construction
  line L126 (52.7225, 52.8686) -> (46.7177, 52.8686) construction
  line L127 (46.7177, 52.8686) -> (46.7177, 42.2853) construction
  line L128 (63.3865, 42.2853) -> (69.0399, 42.2853) construction
  line L129 (69.0399, 42.2853) -> (69.0399, 52.8686) construction
  line L130 (69.0399, 52.8686) -> (63.3865, 52.8686) construction
  line L131 (63.3865, 52.8686) -> (63.3865, 42.2853) construction
  line L132 (80.0552, 42.2853) -> (84.7888, 42.2853) construction
  line L133 (84.7888, 42.2853) -> (84.7888, 52.8686) construction
  line L134 (84.7888, 52.8686) -> (80.0552, 52.8686) construction
  line L135 (80.0552, 52.8686) -> (80.0552, 42.2853) construction
  line L136 (-86.6323, 23.7853) -> (-80.6637, 23.7853) construction
  line L137 (-80.6637, 23.7853) -> (-80.6637, 34.3686) construction
  line L138 (-80.6637, 34.3686) -> (-86.6323, 34.3686) construction
  line L139 (-86.6323, 34.3686) -> (-86.6323, 23.7853) construction
  line L140 (-69.9635, 23.7853) -> (-62.8735, 23.7853) construction
  line L141 (-62.8735, 23.7853) -> (-62.8735, 34.3686) construction
  line L142 (-62.8735, 34.3686) -> (-69.9635, 34.3686) construction
  line L143 (-69.9635, 34.3686) -> (-69.9635, 23.7853) construction
  line L144 (-53.2948, 23.7853) -> (-46.5975, 23.7853) construction
  line L145 (-46.5975, 23.7853) -> (-46.5975, 34.3686) construction
  line L146 (-46.5975, 34.3686) -> (-53.2948, 34.3686) construction
  line L147 (-53.2948, 34.3686) -> (-53.2948, 23.7853) construction
  line L148 (-36.626, 23.7853) -> (-30.6833, 23.7853) construction
  line L149 (-30.6833, 23.7853) -> (-30.6833, 34.3686) construction
  line L150 (-30.6833, 34.3686) -> (-36.626, 34.3686) construction
  line L151 (-36.626, 34.3686) -> (-36.626, 23.7853) construction
  line L152 (-19.9573, 23.7853) -> (-12.8673, 23.7853) construction
  line L153 (-12.8673, 23.7853) -> (-12.8673, 34.3686) construction
  line L154 (-12.8673, 34.3686) -> (-19.9573, 34.3686) construction
  line L155 (-19.9573, 34.3686) -> (-19.9573, 23.7853) construction
  line L156 (-3.2885, 23.7853) -> (2.4941, 23.7853) construction
  line L157 (2.4941, 23.7853) -> (2.4941, 34.3686) construction
  line L158 (2.4941, 34.3686) -> (-3.2885, 34.3686) construction
  line L159 (-3.2885, 34.3686) -> (-3.2885, 23.7853) construction
  line L160 (13.3802, 23.7853) -> (19.1628, 23.7853) construction
  line L161 (19.1628, 23.7853) -> (19.1628, 34.3686) construction
  line L162 (19.1628, 34.3686) -> (13.3802, 34.3686) construction
  line L163 (13.3802, 34.3686) -> (13.3802, 23.7853) construction
  line L164 (30.049, 23.7853) -> (36.9943, 23.7853) construction
  line L165 (36.9943, 23.7853) -> (36.9943, 34.3686) construction
  line L166 (36.9943, 34.3686) -> (30.049, 34.3686) construction
  line L167 (30.049, 34.3686) -> (30.049, 23.7853) construction
  line L168 (46.7177, 23.7853) -> (53.6475, 23.7853) construction
  line L169 (53.6475, 23.7853) -> (53.6475, 34.3686) construction
  line L170 (53.6475, 34.3686) -> (46.7177, 34.3686) construction
  line L171 (46.7177, 34.3686) -> (46.7177, 23.7853) construction
  line L172 (63.3865, 23.7853) -> (70.6315, 23.7853) construction
  line L173 (70.6315, 23.7853) -> (70.6315, 34.3686) construction
  line L174 (70.6315, 34.3686) -> (63.3865, 34.3686) construction
  line L175 (63.3865, 34.3686) -> (63.3865, 23.7853) construction
  line L176 (80.0552, 23.7853) -> (86.7318, 23.7853) construction
  line L177 (86.7318, 23.7853) -> (86.7318, 34.3686) construction
  line L178 (86.7318, 34.3686) -> (80.0552, 34.3686) construction
  line L179 (80.0552, 34.3686) -> (80.0552, 23.7853) construction
  line L180 (-86.6323, 5.2853) -> (-80.6895, 5.2853) construction
  line L181 (-80.6895, 5.2853) -> (-80.6895, 15.8686) construction
  line L182 (-80.6895, 15.8686) -> (-86.6323, 15.8686) construction
  line L183 (-86.6323, 15.8686) -> (-86.6323, 5.2853) construction
  line L184 (-69.9635, 5.2853) -> (-62.8735, 5.2853) construction
  line L185 (-62.8735, 5.2853) -> (-62.8735, 15.8686) construction
  line L186 (-62.8735, 15.8686) -> (-69.9635, 15.8686) construction
  line L187 (-69.9635, 15.8686) -> (-69.9635, 5.2853) construction
  line L188 (-53.2948, 5.2853) -> (-48.5612, 5.2853) construction
  line L189 (-48.5612, 5.2853) -> (-48.5612, 15.8686) construction
  line L190 (-48.5612, 15.8686) -> (-53.2948, 15.8686) construction
  line L191 (-53.2948, 15.8686) -> (-53.2948, 5.2853) construction
  line L192 (-36.626, 5.2853) -> (-30.9055, 5.2853) construction
  line L193 (-30.9055, 5.2853) -> (-30.9055, 15.8686) construction
  line L194 (-30.9055, 15.8686) -> (-36.626, 15.8686) construction
  line L195 (-36.626, 15.8686) -> (-36.626, 5.2853) construction
  line L196 (-19.9573, 5.2853) -> (-18.9548, 5.2853) construction
  line L197 (-18.9548, 5.2853) -> (-18.9548, 15.8686) construction
  line L198 (-18.9548, 15.8686) -> (-19.9573, 15.8686) construction
  line L199 (-19.9573, 15.8686) -> (-19.9573, 5.2853) construction
  line L200 (-3.2885, 5.2853) -> (3.3881, 5.2853) construction
  line L201 (3.3881, 5.2853) -> (3.3881, 15.8686) construction
  line L202 (3.3881, 15.8686) -> (-3.2885, 15.8686) construction
  line L203 (-3.2885, 15.8686) -> (-3.2885, 5.2853) construction
  line L204 (13.3802, 5.2853) -> (19.385, 5.2853) construction
  line L205 (19.385, 5.2853) -> (19.385, 15.8686) construction
  line L206 (19.385, 15.8686) -> (13.3802, 15.8686) construction
  line L207 (13.3802, 15.8686) -> (13.3802, 5.2853) construction
  line L208 (30.049, 5.2853) -> (35.9917, 5.2853) construction
  line L209 (35.9917, 5.2853) -> (35.9917, 15.8686) construction
  line L210 (35.9917, 15.8686) -> (30.049, 15.8686) construction
  line L211 (30.049, 15.8686) -> (30.049, 5.2853) construction
  line L212 (46.7177, 5.2853) -> (52.9809, 5.2853) construction
  line L213 (52.9809, 5.2853) -> (52.9809, 15.8686) construction
  line L214 (52.9809, 15.8686) -> (46.7177, 15.8686) construction
  line L215 (46.7177, 15.8686) -> (46.7177, 5.2853) construction
  line L216 (63.3865, 5.2853) -> (70.4765, 5.2853) construction
  line L217 (70.4765, 5.2853) -> (70.4765, 15.8686) construction
  line L218 (70.4765, 15.8686) -> (63.3865, 15.8686) construction
  line L219 (63.3865, 15.8686) -> (63.3865, 5.2853) construction
  line L220 (80.0552, 5.2853) -> (87.0005, 5.2853) construction
  line L221 (87.0005, 5.2853) -> (87.0005, 15.8686) construction
  line L222 (87.0005, 15.8686) -> (80.0552, 15.8686) construction
  line L223 (80.0552, 15.8686) -> (80.0552, 5.2853) construction
  line L224 (-86.6323, -13.2147) -> (-80.3691, -13.2147) construction
  line L225 (-80.3691, -13.2147) -> (-80.3691, -2.6314) construction
  line L226 (-80.3691, -2.6314) -> (-86.6323, -2.6314) construction
  line L227 (-86.6323, -2.6314) -> (-86.6323, -13.2147) construction
  line L228 (-69.9635, -13.2147) -> (-63.2869, -13.2147) construction
  line L229 (-63.2869, -13.2147) -> (-63.2869, -2.6314) construction
  line L230 (-63.2869, -2.6314) -> (-69.9635, -2.6314) construction
  line L231 (-69.9635, -2.6314) -> (-69.9635, -13.2147) construction
  line L232 (-53.2948, -13.2147) -> (-47.3055, -13.2147) construction
  line L233 (-47.3055, -13.2147) -> (-47.3055, -2.6314) construction
  line L234 (-47.3055, -2.6314) -> (-53.2948, -2.6314) construction
  line L235 (-53.2948, -2.6314) -> (-53.2948, -13.2147) construction
  line L236 (-36.626, -13.2147) -> (-26.885, -13.2147) construction
  line L237 (-26.885, -13.2147) -> (-26.885, -2.6314) construction
  line L238 (-26.885, -2.6314) -> (-36.626, -2.6314) construction
  line L239 (-36.626, -2.6314) -> (-36.626, -13.2147) construction
  line L240 (-19.9573, -13.2147) -> (-12.7123, -13.2147) construction
  line L241 (-12.7123, -13.2147) -> (-12.7123, -2.6314) construction
  line L242 (-12.7123, -2.6314) -> (-19.9573, -2.6314) construction
  line L243 (-19.9573, -2.6314) -> (-19.9573, -13.2147) construction
  line L244 (-3.2885, -13.2147) -> (1.445, -13.2147) construction
  line L245 (1.445, -13.2147) -> (1.445, -2.6314) construction
  line L246 (1.445, -2.6314) -> (-3.2885, -2.6314) construction
  line L247 (-3.2885, -2.6314) -> (-3.2885, -13.2147) construction
  line L248 (13.3802, -13.2147) -> (18.491, -13.2147) construction
  line L249 (18.491, -13.2147) -> (18.491, -2.6314) construction
  line L250 (18.491, -2.6314) -> (13.3802, -2.6314) construction
  line L251 (13.3802, -2.6314) -> (13.3802, -13.2147) construction
  line L252 (30.049, -13.2147) -> (36.0073, -13.2147) construction
  line L253 (36.0073, -13.2147) -> (36.0073, -2.6314) construction
  line L254 (36.0073, -2.6314) -> (30.049, -2.6314) construction
  line L255 (30.049, -2.6314) -> (30.049, -13.2147) construction
  line L256 (46.7177, -13.2147) -> (52.6863, -13.2147) construction
  line L257 (52.6863, -13.2147) -> (52.6863, -2.6314) construction
  line L258 (52.6863, -2.6314) -> (46.7177, -2.6314) construction
  line L259 (46.7177, -2.6314) -> (46.7177, -13.2147) construction
  line L260 (63.3865, -13.2147) -> (68.4973, -13.2147) construction
  line L261 (68.4973, -13.2147) -> (68.4973, -2.6314) construction
  line L262 (68.4973, -2.6314) -> (63.3865, -2.6314) construction
  line L263 (63.3865, -2.6314) -> (63.3865, -13.2147) construction
  line L264 (80.0552, -13.2147) -> (87.0005, -13.2147) construction
  line L265 (87.0005, -13.2147) -> (87.0005, -2.6314) construction
  line L266 (87.0005, -2.6314) -> (80.0552, -2.6314) construction
  line L267 (80.0552, -2.6314) -> (80.0552, -13.2147) construction
  line L268 (-86.6323, -31.7147) -> (-80.643, -31.7147) construction
  line L269 (-80.643, -31.7147) -> (-80.643, -21.1314) construction
  line L270 (-80.643, -21.1314) -> (-86.6323, -21.1314) construction
  line L271 (-86.6323, -21.1314) -> (-86.6323, -31.7147) construction
  line L272 (-69.9635, -31.7147) -> (-64.3101, -31.7147) construction
  line L273 (-64.3101, -31.7147) -> (-64.3101, -21.1314) construction
  line L274 (-64.3101, -21.1314) -> (-69.9635, -21.1314) construction
  line L275 (-69.9635, -21.1314) -> (-69.9635, -31.7147) construction
  line L276 (-53.2948, -31.7147) -> (-47.352, -31.7147) construction
  line L277 (-47.352, -31.7147) -> (-47.352, -21.1314) construction
  line L278 (-47.352, -21.1314) -> (-53.2948, -21.1314) construction
  line L279 (-53.2948, -21.1314) -> (-53.2948, -31.7147) construction
  line L280 (-36.626, -31.7147) -> (-30.6574, -31.7147) construction
  line L281 (-30.6574, -31.7147) -> (-30.6574, -21.1314) construction
  line L282 (-30.6574, -21.1314) -> (-36.626, -21.1314) construction
  line L283 (-36.626, -21.1314) -> (-36.626, -31.7147) construction
  line L284 (-19.9573, -31.7147) -> (-14.3039, -31.7147) construction
  line L285 (-14.3039, -31.7147) -> (-14.3039, -21.1314) construction
  line L286 (-14.3039, -21.1314) -> (-19.9573, -21.1314) construction
  line L287 (-19.9573, -21.1314) -> (-19.9573, -31.7147) construction